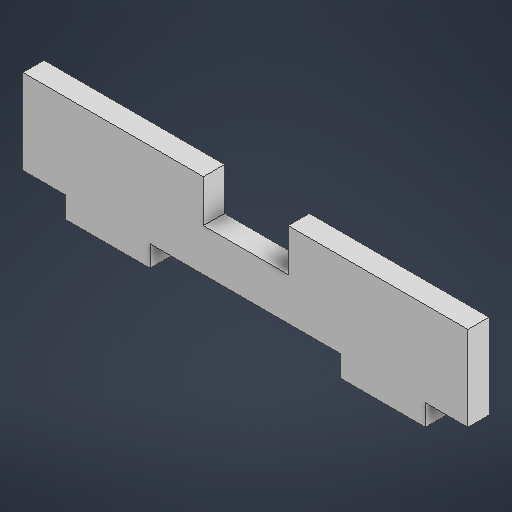
# Autodesk Inventor part: inslide3
Saved by Autodesk Inventor 2026.2 (Build 302298000, 298)
## iProperties
Created: 2026-04-17
Part Number: inslide3
Material: Generic
Document SubType Name: Modeling
Designer: danda
Density: 1 g/cm^3
Appearance: Default
Author: danda
Autodesk Inventor part; units mm, degrees
ref_plane "YZ Plane" through (0, 0, 0) normal (1, 0, 0) x (0, 1, 0)
ref_plane "XZ Plane" through (0, 0, 0) normal (0, 1, 0) x (-1, 0, 0)
ref_plane "XY Plane" through (0, 0, 0) normal (0, 0, 1) x (1, 0, 0)
sketch "Sketch1" plane through (0, 0, 0) normal (0, 0, 1) x (1, 0, 0)
  line L0 (23.0237, 36.3892) -> (128.0237, 36.3892)
  line L1 (128.0237, 36.3892) -> (128.0237, 16.3892)
  line L2 (128.0237, 16.3892) -> (23.0237, 16.3892)
  line L3 (23.0237, 16.3892) -> (23.0237, 36.3892)
  line L4 (33.0237, 16.3892) -> (53.0237, 16.3892)
  line L5 (53.0237, 16.3892) -> (53.0237, 11.3892)
  line L6 (53.0237, 11.3892) -> (33.0237, 11.3892)
  line L7 (33.0237, 11.3892) -> (33.0237, 16.3892)
  line L8 (98.0237, 16.3892) -> (118.0237, 16.3892)
  line L9 (118.0237, 16.3892) -> (118.0237, 11.3892)
  line L10 (118.0237, 11.3892) -> (98.0237, 11.3892)
  line L11 (98.0237, 11.3892) -> (98.0237, 16.3892)
  point P0 (0, 0)
  point P1 (33.0237, 13.8892)
  dimension "d0" = 105
  dimension "d1" = 20
  dimension "d2" = 20
  dimension "d3" = 5
  dimension "d4" = 20
  dimension "d5" = 5
  dimension "d6" = 10
  dimension "d7" = 10
  constraints: 24 end point, 6 parallel, 3 horizontal, 3 perpendicular, 2 point on line, 1 midpoint
  measures "d0" distance of L1.end L2.end
  measures "d1" distance of L0.end L1.end
  measures "d2" distance of L5.end L6.end
  measures "d3" distance of L4.end L5.end
  measures "d4" distance of L9.end L10.end
  measures "d5" distance of L8.end L9.end
  measures "d6" horizontal distance of L2.end point (33.024, 13.889)
  measures "d7" distance from line of L9 L1.end
extrude "Extrusion1" add sketch "Sketch1" along normal blind 5
sketch "Sketch2" plane through (0, 0, 5) normal (0, 0, 1) x (1, 0, 0)
  line L0 (128.0237, 36.3892) -> (23.0237, 36.3892) projected
  line L1 (65.6129, 36.3892) -> (85.6129, 36.3892)
  line L2 (85.6129, 36.3892) -> (85.6129, 26.3892)
  line L3 (85.6129, 26.3892) -> (65.6129, 26.3892)
  line L4 (65.6129, 26.3892) -> (65.6129, 36.3892)
  point P0 (0, 0)
  dimension "d10" = 20
  dimension "d11" = 10
  constraints: 8 end point, 2 parallel, 1 horizontal, 1 perpendicular, 1 point on line
  measures "d10" distance of L2.end L3.end
  measures "d11" distance of L1.end L2.end
extrude "Extrusion2" cut sketch "Sketch2" against normal blind 10
body "Solid1"
